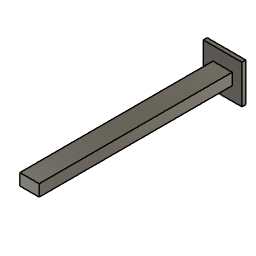
Cantilever Beam (Autodesk Fusion 360 design; units mm, degrees)
Autodesk Fusion 360 part; units mm, degrees
sketch "Sketch1" plane through (0, 0, 0) normal (0, 1, 0) x (1, 0, 0)
  line L0 (500, 500) -> (-500, 500)
  line L1 (-500, 500) -> (-500, -500)
  line L2 (-500, -500) -> (500, -500)
  line L3 (500, -500) -> (500, 500)
  line L4 (500, 500) -> (-500, -500) construction
  line L5 (-500, 500) -> (500, -500) construction
  dimension "d1" = 1000
  dimension "d2" = 1000
  constraint horizontal L0
  constraint perpendicular L0 L1
  constraint parallel L0 L2
  constraint parallel L1 L3
  constraint coincident L4 origin
  constraint coincident L5 origin
  measures "d1" distance of L1.end L2.end
  measures "d2" distance of L0.end L1.end
extrude "Extrude1" add sketch "Sketch1" along normal blind 100 makes body 1 in component "WALL"
sketch "Sketch2" plane through (0, 0, 0) normal (0, -1, 0) x (1, 0, 0)
  line L0 (500, -500) -> (500, 500)
  line L1 (500, 500) -> (-500, 500)
  line L2 (-500, 500) -> (-500, -500)
  line L3 (-500, -500) -> (500, -500)
  line L4 (250, -150) -> (-250, -150)
  line L5 (-250, -150) -> (-250, 150)
  line L6 (-250, 150) -> (250, 150)
  line L7 (250, 150) -> (250, -150)
  line L8 (250, -150) -> (-250, 150) construction
  line L9 (-250, -150) -> (250, 150) construction
  constraint horizontal L4
  constraint perpendicular L4 L5
  constraint parallel L4 L6
  constraint parallel L5 L7
  constraint coincident L8 origin
  constraint coincident L9 origin
extrude "Extrude1'" add sketch "Sketch2" along normal blind 5000 separate body contours L4 L5 L6 L7 makes body 2 in component "BEAM"
component "WALL" placed x (1, 0, 0) y (0, 1, 0) z (0, 0, 1) at (0, 0, 0)
component "BEAM" placed x (1, 0, 0) y (0, 1, 0) z (0, 0, 1) at (0, 0, 0)
